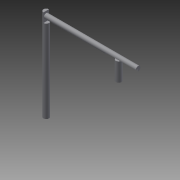
# Autodesk Inventor part: shaft1
Saved by Autodesk Inventor 2015 (Build 190159000, 159)
## iProperties
Created: 2020-01-21
Part Number: shaft1
Material: Generic
Document SubType Name: Modeling
Designer: hp
Density: 1 g/cm^3
Appearance: Default
Author: hp
Autodesk Inventor part; units mm, degrees
ref_plane "YZ Plane" through (0, 0, 0) normal (1, 0, 0) x (0, 1, 0)
ref_plane "XZ Plane" through (0, 0, 0) normal (0, 1, 0) x (-1, 0, 0)
ref_plane "XY Plane" through (0, 0, 0) normal (0, 0, 1) x (1, 0, 0)
sketch "Sketch1" plane through (0, 0, 0) normal (0, 1, 0) x (-1, 0, 0)
  circle A0 centre (0, 0) radius 22.86
  dimension "d0" = 45.72
  constraints: 1 centre point, 1 coincident
  measures "d0" diameter of A0
extrude "Extrusion1" add sketch "Sketch1" along normal blind 762
sketch "Sketch2" plane through (0, 762, 0) normal (0, 1, 0) x (1, 0, 0)
  circle A0 centre (0, 0) radius 22.86 projected
  line L0 (0, 22.86) -> (28.6058, 22.86)
  line L1 (28.6058, 22.86) -> (28.6058, -22.86)
  line L2 (28.6058, -22.86) -> (0, -22.86)
  line L3 (0, -22.86) -> (0, 22.86)
  constraints: 8 end point, 2 parallel, 1 horizontal, 1 perpendicular, 1 vertical alignment, 1 other
extrude "Extrusion2" cut sketch "Sketch2" against normal blind 76.2 contours A0 L3 | A0 L0 L1 L2 picked at (10.9262, 0.7546)
sketch "Sketch3" plane through (0, 762, 22.86) normal (1, 0, 0) x (0, 0, -1)
  circle A0 centre (22.86, -35.2146) radius 19.5985
  point P0 (22.86, -762)
  constraints: 1 centre point
extrude "Extrusion3" add sketch "Sketch3" along normal blind 762
sketch "Sketch4" plane through (762, 726.7854, 0) normal (1, 0, 0) x (0, 0, -1)
  line L0 (-22.86, -40.9854) -> (-22.86, 35.2146) projected
  line L1 (0, 0) -> (-22.86, 0)
  line L2 (-22.86, 0) -> (-22.86, -25.8256)
  line L3 (-22.86, -25.8256) -> (0, -25.8256)
  line L4 (0, -25.8256) -> (0, 0)
  point P0 (0, -726.7854)
  constraints: 8 end point, 2 parallel, 1 horizontal, 1 perpendicular, 1 point on line
extrude "Extrusion4" cut sketch "Sketch4" against normal blind 254
sketch "Sketch5" plane through (762, 726.7854, 0) normal (0, -1, 0) x (1, 0, 0)
  line L0 (0, 0) -> (-148.3868, 0)
  line L1 (0, 0) -> (-254, 0) projected
  circle A0 centre (-148.3868, 12.7759) radius 22.86
  point P0 (-762, 0)
  dimension "d9" = 148.3868
  dimension "d13" = 45.72
  constraints: 2 end point, 1 centre point, 1 point on line
  measures "d9" distance of L0.start L0.end
  measures "d13" diameter of A0
extrude "Extrusion5" add sketch "Sketch5" along normal blind 152.4
body "Solid1"
